Encoder Magnet holder_v1 (Autodesk Fusion 360 design; units mm, degrees)
Autodesk Fusion 360 part; units mm, degrees
sketch "Sketch1" plane through (0, 0, 0) normal (0, 0, 1) x (1, 0, 0)
  circle A0 centre (0, 0) radius 5
  circle A1 centre (0, 0) radius 1.65
  dimension "d1" = 10
  dimension "d2" = 3.3
  constraint coincident A0.centre A1.centre
  measures "d1" diameter of A0
  measures "d2" diameter of A1
extrude "Extrude1" add sketch "Sketch1" along normal blind 1
sketch "Sketch2" plane through (0, 0, 1) normal (0, 0, 1) x (-1, 0, 0)
  circle A0 centre (0, 0) radius 1.65
  circle A1 centre (0, 0) radius 5
  circle A2 centre (0, 0) radius 3.075
  dimension "d5" = 6.15
  constraint coincident A0.centre A1.centre
  measures "d5" diameter of A2
extrude "Extrude2" add sketch "Sketch2" along normal blind 8.8 contours A1
sketch "Sketch3" plane through (0, 0, 0) normal (0, 0, -1) x (1, 0, 0)
  circle A0 centre (0, 0) radius 1.65
  circle A1 centre (0, 0) radius 5
  circle A2 centre (0, 0) radius 4
  dimension "d8" = 8
  constraint coincident A0.centre A1.centre
  measures "d8" diameter of A2
extrude "Extrude3" add sketch "Sketch3" along normal blind 0.5 contours A2
sketch "Sketch4" plane through (0, 0, 0) normal (0, 1, 0) x (1, 0, 0)
  ellipse E0 centre (0, -9.8) end of major axis (-1, -9.8) minor radius 5
  line L0 (1, -9.8) -> (-1, -9.8)
  line L1 (0, -4.8) -> (0, -14.8)
  line L2 (-5, -9.8) -> (5, -9.8)
  line L3 (-5, 0) -> (5, 0)
  dimension "d11" = 2
  dimension "d12" = 10
  dimension "d15" = 9.8
  dimension "d16" = 9.8
  constraint coincident E0 L0.start
  constraint coincident E0 L0.end
  constraint coincident E0 L1.start
  constraint coincident E0 L1.end
  constraint horizontal L0
  measures "d11" distance of E0
  measures "d15" distance of origin E0.centre
  measures "d16" distance of L2 L3
extrude "Extrude4" cut sketch "Sketch4" against normal blind 15
equation "d2 = 3 mm + 0.3 mm"
equation "d15 = d16"
